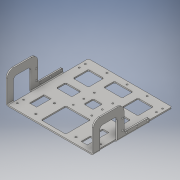
# Autodesk Inventor part: BadanAtasRevisi
Saved by Autodesk Inventor 2016 (Build 200138000, 138)
## iProperties
Created: 2017-04-23
Part Number: BadanAtasRevisi
Material: Generic
Document SubType Name: Modeling
Designer: Ghana
Density: 1 g/cm^3
Appearance: Default
Author: Ghana
Autodesk Inventor part; units mm, degrees
note: some values were not read from the file. Chosen so that the rebuilt part matches the saved one: bend side of "Bend Part6".
ref_plane "YZ Plane" through (0, 0, 0) normal (1, 0, 0) x (0, 1, 0)
ref_plane "XZ Plane" through (0, 0, 0) normal (0, 1, 0) x (-1, 0, 0)
ref_plane "XY Plane" through (0, 0, 0) normal (0, 0, 1) x (1, 0, 0)
sketch "Sketch1" plane through (0, 0, 0) normal (0, 1, 0) x (-1, 0, 0)
  circle A0 centre (82.5, -70) radius 1.3
  circle A1 centre (82.5, -53) radius 1.3
  circle A2 centre (82.5, -87) radius 1.3
  circle A3 centre (100, -125.0019) radius 1.3
  circle A4 centre (35, -125.0019) radius 1.3
  circle A5 centre (52.5, -70) radius 1.3
  circle A6 centre (52.5, -53) radius 1.3
  circle A7 centre (52.5, -87) radius 1.3
  line L0 (85.5, -45.7826) -> (49.5, -45.7826)
  line L1 (47.5, -43.7826) -> (47.5, -7.7826)
  line L2 (49.5, -5.7826) -> (85.5, -5.7826)
  line L3 (87.5, -7.7826) -> (87.5, -43.7826)
  arc A8 (85.5, -45.7826) -> (87.5, -43.7826) centre (85.5, -43.7826) ccw
  arc A9 (47.5, -43.7826) -> (49.5, -45.7826) centre (49.5, -43.7826) ccw
  arc A10 (49.5, -5.7826) -> (47.5, -7.7826) centre (49.5, -7.7826) ccw
  arc A11 (87.5, -7.7826) -> (85.5, -5.7826) centre (85.5, -7.7826) ccw
  line L4 (118, -115) -> (97, -115)
  line L5 (95, -113) -> (95, -92)
  line L6 (97, -90) -> (118, -90)
  line L7 (120, -92) -> (120, -113)
  arc A12 (118, -115) -> (120, -113) centre (118, -113) ccw
  arc A13 (95, -113) -> (97, -115) centre (97, -113) ccw
  arc A14 (97, -90) -> (95, -92) centre (97, -92) ccw
  arc A15 (120, -92) -> (118, -90) centre (118, -92) ccw
  line L8 (17, -115) -> (38, -115)
  line L9 (40, -113) -> (40, -92)
  line L10 (38, -90) -> (17, -90)
  line L11 (15, -92) -> (15, -113)
  arc A16 (15, -113) -> (17, -115) centre (17, -113) ccw
  arc A17 (38, -115) -> (40, -113) centre (38, -113) ccw
  arc A18 (40, -92) -> (38, -90) centre (38, -92) ccw
  arc A19 (17, -90) -> (15, -92) centre (17, -92) ccw
  line L12 (118, -78) -> (97, -78)
  line L13 (95, -76) -> (95, -65)
  line L14 (97, -63) -> (118, -63)
  line L15 (120, -65) -> (120, -76)
  arc A20 (118, -78) -> (120, -76) centre (118, -76) ccw
  arc A21 (95, -76) -> (97, -78) centre (97, -76) ccw
  arc A22 (97, -63) -> (95, -65) centre (97, -65) ccw
  arc A23 (120, -65) -> (118, -63) centre (118, -65) ccw
  line L16 (17, -78) -> (38, -78)
  line L17 (40, -76) -> (40, -65)
  line L18 (38, -63) -> (17, -63)
  line L19 (15, -65) -> (15, -76)
  arc A24 (15, -76) -> (17, -78) centre (17, -76) ccw
  arc A25 (38, -78) -> (40, -76) centre (38, -76) ccw
  arc A26 (40, -65) -> (38, -63) centre (38, -65) ccw
  arc A27 (17, -63) -> (15, -65) centre (17, -65) ccw
  circle A28 centre (100, -40) radius 1.55
  circle A29 centre (100, -10) radius 1.55
  circle A30 centre (35, -40) radius 1.55
  circle A31 centre (35, -10) radius 1.55
  line L20 (120.5, -43.5) -> (109, -43.5)
  line L21 (109, -43.5) -> (109, -20)
  line L22 (109, -20) -> (120.5, -20)
  line L23 (120.5, -20) -> (120.5, -43.5)
  line L24 (15, -43) -> (25, -43)
  line L25 (25, -43) -> (25, -28)
  line L26 (25, -28) -> (15, -28)
  line L27 (15, -28) -> (15, -43)
  line L28 (25, -23) -> (15, -23)
  line L29 (15, -23) -> (15, -8)
  line L30 (15, -8) -> (25, -8)
  line L31 (25, -8) -> (25, -23)
  line L32 (0, 0) -> (135, 0)
  line L33 (135, 0) -> (135, -128)
  line L34 (133, -130) -> (2, -130)
  line L35 (0, -128) -> (0, 0)
  line L36 (62, -62.5) -> (73, -62.5)
  line L37 (75, -64.5) -> (75, -75.5)
  line L38 (73, -77.5) -> (62, -77.5)
  line L39 (60, -75.5) -> (60, -64.5)
  arc A32 (73, -77.5) -> (75, -75.5) centre (73, -75.5) ccw
  arc A33 (60, -75.5) -> (62, -77.5) centre (62, -75.5) ccw
  arc A34 (62, -62.5) -> (60, -64.5) centre (62, -64.5) ccw
  arc A35 (75, -64.5) -> (73, -62.5) centre (73, -64.5) ccw
  circle A36 centre (130, -10) radius 1.3
  circle A37 centre (130, -20) radius 1.3
  circle A38 centre (130, -120) radius 1.3
  circle A39 centre (130, -110) radius 1.3
  line L40 (135, 0) -> (137, 0)
  line L41 (137, 0) -> (137, -10)
  line L42 (137, -90) -> (135, -90)
  line L43 (135, -90) -> (135, 0)
  circle A40 centre (67.5, -125.0019) radius 1.3
  circle A41 centre (139.8, -87) radius 1.3
  circle A42 centre (139.8, -70) radius 1.3
  circle A43 centre (139.8, -53) radius 1.3
  circle A44 centre (146.3, -46.7) radius 1.3
  circle A45 centre (163.3, -46.7) radius 1.3
  line L44 (137, -90) -> (140.4, -90)
  line L45 (142.4, -50.3) -> (142.4, -88)
  line L46 (143.4, -49.3) -> (172.4, -49.3)
  line L47 (182.4, -39.3) -> (182.4, -10)
  line L48 (172.4, 0) -> (137, 0)
  arc A46 (172.4, -49.3) -> (182.4, -39.3) centre (172.4, -39.3) ccw
  arc A47 (182.4, -10) -> (172.4, 0) centre (172.4, -10) ccw
  arc A48 (143.4, -49.3) -> (142.4, -50.3) centre (143.4, -50.3) ccw
  arc A49 (140.4, -90) -> (142.4, -88) centre (140.4, -88) ccw
  arc A50 (133, -130) -> (135, -128) centre (133, -128) ccw
  arc A51 (0, -128) -> (2, -130) centre (2, -128) ccw
  circle A52 centre (5, -10) radius 1.3
  circle A53 centre (5, -20) radius 1.3
  circle A54 centre (5, -120) radius 1.3
  circle A55 centre (5, -110) radius 1.3
  line L49 (0, 0) -> (-2, 0)
  line L50 (-2, 0) -> (-2, -10)
  line L51 (-2, -90) -> (0, -90)
  line L52 (0, -90) -> (0, 0)
  circle A56 centre (-4.8, -87) radius 1.3
  circle A57 centre (-4.8, -70) radius 1.3
  circle A58 centre (-4.8, -53) radius 1.3
  circle A59 centre (-11.3, -46.7) radius 1.3
  circle A60 centre (-28.3, -46.7) radius 1.3
  line L53 (-2, -90) -> (-5.4, -90)
  line L54 (-7.4, -50.3) -> (-7.4, -88)
  line L55 (-8.4, -49.3) -> (-37.4, -49.3)
  line L56 (-47.4, -39.3) -> (-47.4, -10)
  line L57 (-37.4, 0) -> (-2, 0)
  arc A61 (-47.4, -39.3) -> (-37.4, -49.3) centre (-37.4, -39.3) ccw
  arc A62 (-37.4, 0) -> (-47.4, -10) centre (-37.4, -10) ccw
  arc A63 (-7.4, -50.3) -> (-8.4, -49.3) centre (-8.4, -50.3) ccw
  arc A64 (-7.4, -88) -> (-5.4, -90) centre (-5.4, -88) ccw
  line L58 (54.5, -102) -> (80.5, -102)
  line L59 (82.5, -104) -> (82.5, -117.5)
  line L60 (80.5, -119.5) -> (54.5, -119.5)
  line L61 (52.5, -117.5) -> (52.5, -104)
  arc A65 (80.5, -119.5) -> (82.5, -117.5) centre (80.5, -117.5) ccw
  arc A66 (52.5, -117.5) -> (54.5, -119.5) centre (54.5, -117.5) ccw
  arc A67 (54.5, -102) -> (52.5, -104) centre (54.5, -104) ccw
  arc A68 (82.5, -104) -> (80.5, -102) centre (80.5, -104) ccw
  line L62 (67.5, 0) -> (67.5, -34.0355)
  line L63 (135, -10) -> (165, -10)
  line L64 (170, -15) -> (170, -33)
  line L65 (165, -38) -> (135, -38)
  line L66 (135, -38) -> (135, -10)
  arc A69 (165, -38) -> (170, -33) centre (165, -33) ccw
  arc A70 (170, -15) -> (165, -10) centre (165, -15) ccw
  line L67 (137, -38) -> (137, -90)
  line L68 (0, -10) -> (-30, -10)
  line L69 (-35, -15) -> (-35, -33)
  line L70 (-30, -38) -> (0, -38)
  line L71 (0, -38) -> (0, -10)
  arc A71 (-35, -33) -> (-30, -38) centre (-30, -33) ccw
  arc A72 (-30, -10) -> (-35, -15) centre (-30, -15) ccw
  line L72 (-2, -38) -> (-2, -90)
  point P0 (47.5, -5.7826)
  point P1 (47.5, -45.7826)
  point P2 (87.5, -5.7826)
  point P3 (95, -90)
  point P4 (95, -115)
  point P5 (120, -90)
  point P6 (40, -90)
  point P7 (40, -115)
  point P8 (15, -90)
  point P9 (95, -63)
  point P10 (95, -78)
  point P11 (120, -63)
  point P12 (40, -63)
  point P13 (40, -78)
  point P14 (15, -63)
  point P15 (135, -130)
  point P16 (0, -130)
  point P17 (75, -77.5)
  point P18 (75, -62.5)
  point P19 (60, -77.5)
  point P20 (142.4, -49.3)
  point P21 (182.4, -49.3)
  point P22 (-7.4, -49.3)
  point P23 (-47.4, -49.3)
  point P24 (52.5, -102)
  point P25 (82.5, -119.5)
  point P26 (82.5, -102)
  point P27 (170, -38)
  point P28 (170, -10)
  dimension "d28" = 40
  dimension "d29" = 40
  dimension "d30" = 2
  dimension "d33" = 25
  dimension "d34" = 25
  dimension "d52" = 25
  dimension "d53" = 15
  dimension "d61" = 3.1
  dimension "d65" = 11.5
  dimension "d66" = 23.5
  dimension "d70" = 15
  dimension "d71" = 5
  dimension "d72" = 15
  dimension "d115" = 135
  dimension "d116" = 130
  dimension "d117" = 15
  dimension "d118" = 15
  dimension "d119" = 2
  dimension "d122" = 2.6
  dimension "d128" = 2
  dimension "d129" = 10
  dimension "d130" = 2.6
  dimension "d131" = 32.5
  dimension "d132" = 32.5
  dimension "d133" = 65
  dimension "d134" = 30
  dimension "d136" = 2.6
  dimension "d141" = 6.5
  dimension "d143" = 17
  dimension "d144" = 6.3
  dimension "d145" = 17
  dimension "d146" = 17
  dimension "d149" = 40
  dimension "d153" = 10
  dimension "d155" = 1
  dimension "d156" = 2
  dimension "d157" = 2
  dimension "d159" = 15
  dimension "d160" = 17.5
  dimension "d161" = 2
  dimension "d175" = 35
  dimension "d176" = 28
  dimension "d177" = 5
  constraints: 146 end point, 84 point on circle, 73 centre point, 63 point on line, 56 tangent, 32 equal radius, 23 parallel, 14 perpendicular, 13 horizontal, 8 symmetric about line, 5 vertical alignment, 1 horizontal alignment, 1 midpoint, 1 vertical, 2 other
  measures "d28" distance of point (47.5, -5.783) point (87.5, -5.783)
  measures "d29" distance of point (47.5, -45.783) point (47.5, -5.783)
  measures "d30" radius of A8
  measures "d33" distance of point (95, -90) point (120, -90)
  measures "d34" distance of point (95, -115) point (95, -90)
  measures "d52" distance of point (95, -63) point (120, -63)
  measures "d53" distance of point (95, -78) point (95, -63)
  measures "d61" diameter of A28
  measures "d65" distance of L21.end L22.end
  measures "d66" distance of L20.end L21.end
  measures "d70" distance of L25.end L24.end
  measures "d71" distance of L25.end L28.start
  measures "d72" distance of L28.end L29.end
  measures "d115" distance of point (135, -130) point (0, -130)
  measures "d116" distance of L32.end point (135, -130)
  measures "d117" distance of point (75, -77.5) point (60, -77.5)
  measures "d118" distance of point (75, -62.5) point (75, -77.5)
  measures "d119" radius of A32
  measures "d122" diameter of A36
  measures "d128" distance of L42.start L42.end
  measures "d129" distance of L24.start L24.end
  measures "d130" diameter of A3
  measures "d131" distance of A3.centre A40.centre
  measures "d132" distance of A4.centre A40.centre
  measures "d133" distance of A30.centre A28.centre
  measures "d134" distance of A29.centre A28.centre
  measures "d136" diameter of A41
  measures "d141" horizontal distance of A43.centre A44.centre
  measures "d143" distance of A44.centre A45.centre
  measures "d144" vertical distance of A43.centre A44.centre
  measures "d145" distance of A42.centre A41.centre
  measures "d146" distance of A43.centre A42.centre
  measures "d149" distance of point (142.4, -49.3) point (182.4, -49.3)
  measures "d153" radius of A46
  measures "d155" radius of A48
  measures "d156" radius of A49
  measures "d157" radius of A50
  measures "d159" distance of A7.centre point (52.5, -102)
  measures "d160" distance of point (82.5, -102) point (82.5, -119.5)
  measures "d161" radius of A65
  measures "d175" distance of point (170, -38) L65.end
  measures "d176" distance of point (170, -10) point (170, -38)
  measures "d177" radius of A69
extrude "Extrusion5" add sketch "Sketch1" along normal blind 2 contours L32 L33 A50 L34 A51 L35 | L35 L68 L50 L49 | L50 L68 A72 L69 A71 L70 L72 L53 A64 L54 A63 L55 A61 L56 A62 L57 | L40 L41 L63 L33 | L35 L51 L72 L70 | L48 A47 L47 A46 L46 A48 L45 A49 L44 L67 L65 A69 L64 A70 L63 L41 | L65 L67 L42 L33
sketch "Sketch7" plane through (0, 2, 0) normal (0, 1, 0) x (1, 0, 0)
  arc A0 (-47.5, 43.7826) -> (-49.5, 45.7826) centre (-49.5, 43.7826) ccw projected
  line L0 (-47.5, 43.7826) -> (-47.5, 7.7826) projected
  arc A1 (-49.5, 5.7826) -> (-47.5, 7.7826) centre (-49.5, 7.7826) ccw projected
  line L1 (-49.5, 5.7826) -> (-85.5, 5.7826) projected
  arc A2 (-87.5, 7.7826) -> (-85.5, 5.7826) centre (-85.5, 7.7826) ccw projected
  line L2 (-87.5, 7.7826) -> (-87.5, 43.7826) projected
  arc A3 (-85.5, 45.7826) -> (-87.5, 43.7826) centre (-85.5, 43.7826) ccw projected
  line L3 (-85.5, 45.7826) -> (-49.5, 45.7826) projected
  arc A4 (-15, 113) -> (-17, 115) centre (-17, 113) ccw projected
  line L4 (-15, 113) -> (-15, 92) projected
  arc A5 (-17, 90) -> (-15, 92) centre (-17, 92) ccw projected
  line L5 (-17, 90) -> (-38, 90) projected
  arc A6 (-40, 92) -> (-38, 90) centre (-38, 92) ccw projected
  line L6 (-40, 92) -> (-40, 113) projected
  arc A7 (-38, 115) -> (-40, 113) centre (-38, 113) ccw projected
  line L7 (-38, 115) -> (-17, 115) projected
  arc A8 (-95, 113) -> (-97, 115) centre (-97, 113) ccw projected
  line L8 (-95, 113) -> (-95, 92) projected
  arc A9 (-97, 90) -> (-95, 92) centre (-97, 92) ccw projected
  line L9 (-97, 90) -> (-118, 90) projected
  arc A10 (-120, 92) -> (-118, 90) centre (-118, 92) ccw projected
  line L10 (-120, 92) -> (-120, 113) projected
  arc A11 (-118, 115) -> (-120, 113) centre (-118, 113) ccw projected
  line L11 (-118, 115) -> (-97, 115) projected
  arc A12 (-52.5, 117.5) -> (-54.5, 119.5) centre (-54.5, 117.5) ccw projected
  line L12 (-52.5, 117.5) -> (-52.5, 104) projected
  arc A13 (-54.5, 102) -> (-52.5, 104) centre (-54.5, 104) ccw projected
  line L13 (-54.5, 102) -> (-80.5, 102) projected
  arc A14 (-82.5, 104) -> (-80.5, 102) centre (-80.5, 104) ccw projected
  line L14 (-82.5, 104) -> (-82.5, 117.5) projected
  arc A15 (-80.5, 119.5) -> (-82.5, 117.5) centre (-80.5, 117.5) ccw projected
  line L15 (-80.5, 119.5) -> (-54.5, 119.5) projected
  arc A16 (-38, 78) -> (-40, 76) centre (-38, 76) ccw projected
  line L16 (-38, 78) -> (-17, 78) projected
  arc A17 (-15, 76) -> (-17, 78) centre (-17, 76) ccw projected
  line L17 (-15, 76) -> (-15, 65) projected
  arc A18 (-17, 63) -> (-15, 65) centre (-17, 65) ccw projected
  line L18 (-17, 63) -> (-38, 63) projected
  arc A19 (-40, 65) -> (-38, 63) centre (-38, 65) ccw projected
  line L19 (-40, 65) -> (-40, 76) projected
  arc A20 (-95, 76) -> (-97, 78) centre (-97, 76) ccw projected
  line L20 (-95, 76) -> (-95, 65) projected
  arc A21 (-97, 63) -> (-95, 65) centre (-97, 65) ccw projected
  line L21 (-97, 63) -> (-118, 63) projected
  arc A22 (-120, 65) -> (-118, 63) centre (-118, 65) ccw projected
  line L22 (-120, 65) -> (-120, 76) projected
  arc A23 (-118, 78) -> (-120, 76) centre (-118, 76) ccw projected
  line L23 (-118, 78) -> (-97, 78) projected
  line L24 (-109, 43.5) -> (-109, 20) projected
  line L25 (-109, 20) -> (-120.5, 20) projected
  line L26 (-120.5, 20) -> (-120.5, 43.5) projected
  line L27 (-120.5, 43.5) -> (-109, 43.5) projected
  arc A24 (-60, 75.5) -> (-62, 77.5) centre (-62, 75.5) ccw projected
  line L28 (-60, 75.5) -> (-60, 64.5) projected
  arc A25 (-62, 62.5) -> (-60, 64.5) centre (-62, 64.5) ccw projected
  line L29 (-62, 62.5) -> (-73, 62.5) projected
  arc A26 (-75, 64.5) -> (-73, 62.5) centre (-73, 64.5) ccw projected
  line L30 (-75, 64.5) -> (-75, 75.5) projected
  arc A27 (-73, 77.5) -> (-75, 75.5) centre (-73, 75.5) ccw projected
  line L31 (-73, 77.5) -> (-62, 77.5) projected
  line L32 (-15, 23) -> (-15, 8) projected
  line L33 (-15, 8) -> (-25, 8) projected
  line L34 (-25, 8) -> (-25, 23) projected
  line L35 (-25, 23) -> (-15, 23) projected
  line L36 (-15, 43) -> (-15, 28) projected
  line L37 (-15, 28) -> (-25, 28) projected
  line L38 (-25, 28) -> (-25, 43) projected
  line L39 (-25, 43) -> (-15, 43) projected
  circle A28 centre (-35, 10) radius 1.55 projected
  circle A29 centre (-35, 40) radius 1.55 projected
  circle A30 centre (-100, 10) radius 1.55 projected
  circle A31 centre (-100, 40) radius 1.55 projected
  circle A32 centre (-5, 110) radius 1.3 projected
  circle A33 centre (-5, 120) radius 1.3 projected
  circle A34 centre (-5, 10) radius 1.3 projected
  circle A35 centre (-5, 20) radius 1.3 projected
  circle A36 centre (-67.5, 125.0019) radius 1.3 projected
  circle A37 centre (-130, 110) radius 1.3 projected
  circle A38 centre (-130, 120) radius 1.3 projected
  circle A39 centre (-130, 20) radius 1.3 projected
  circle A40 centre (-130, 10) radius 1.3 projected
  circle A41 centre (-52.5, 70) radius 1.3 projected
  circle A42 centre (-52.5, 53) radius 1.3 projected
  circle A43 centre (-52.5, 87) radius 1.3 projected
  circle A44 centre (-35, 125.0019) radius 1.3 projected
  circle A45 centre (-100, 125.0019) radius 1.3 projected
  circle A46 centre (-82.5, 87) radius 1.3 projected
  circle A47 centre (-82.5, 53) radius 1.3 projected
  circle A48 centre (-82.5, 70) radius 1.3 projected
  circle A49 centre (-163.3, 46.7) radius 1.3 projected
  circle A50 centre (-146.3, 46.7) radius 1.3 projected
  circle A51 centre (-139.8, 53) radius 1.3 projected
  circle A52 centre (-139.8, 70) radius 1.3 projected
  circle A53 centre (-139.8, 87) radius 1.3 projected
  circle A54 centre (28.3, 46.7) radius 1.3 projected
  circle A55 centre (11.3, 46.7) radius 1.3 projected
  circle A56 centre (4.8, 53) radius 1.3 projected
  circle A57 centre (4.8, 70) radius 1.3 projected
  circle A58 centre (4.8, 87) radius 1.3 projected
  line L40 (0, 10) -> (0, 38) projected
  line L41 (0, 38) -> (30, 38) projected
  arc A59 (35, 33) -> (30, 38) centre (30, 33) ccw projected
  line L42 (35, 33) -> (35, 15) projected
  arc A60 (30, 10) -> (35, 15) centre (30, 15) ccw projected
  line L43 (30, 10) -> (0, 10) projected
  line L44 (-135, 10) -> (-165, 10) projected
  arc A61 (-170, 15) -> (-165, 10) centre (-165, 15) ccw projected
  line L45 (-170, 15) -> (-170, 33) projected
  arc A62 (-165, 38) -> (-170, 33) centre (-165, 33) ccw projected
  line L46 (-165, 38) -> (-135, 38) projected
  line L47 (-135, 38) -> (-135, 10) projected
  line L48 (-172.4, 0) -> (37.4, 0) projected
  arc A63 (37.4, 0) -> (47.4, 10) centre (37.4, 10) ccw projected
  line L49 (47.4, 10) -> (47.4, 39.3) projected
  arc A64 (47.4, 39.3) -> (37.4, 49.3) centre (37.4, 39.3) ccw projected
  line L50 (37.4, 49.3) -> (8.4, 49.3) projected
  arc A65 (7.4, 50.3) -> (8.4, 49.3) centre (8.4, 50.3) ccw projected
  line L51 (7.4, 50.3) -> (7.4, 88) projected
  arc A66 (7.4, 88) -> (5.4, 90) centre (5.4, 88) ccw projected
  line L52 (5.4, 90) -> (0, 90) projected
  line L53 (0, 90) -> (0, 128) projected
  arc A67 (0, 128) -> (-2, 130) centre (-2, 128) ccw projected
  line L54 (-2, 130) -> (-133, 130) projected
  arc A68 (-133, 130) -> (-135, 128) centre (-133, 128) ccw projected
  line L55 (-135, 128) -> (-135, 90) projected
  line L56 (-135, 90) -> (-140.4, 90) projected
  arc A69 (-140.4, 90) -> (-142.4, 88) centre (-140.4, 88) ccw projected
  line L57 (-142.4, 88) -> (-142.4, 50.3) projected
  arc A70 (-143.4, 49.3) -> (-142.4, 50.3) centre (-143.4, 50.3) ccw projected
  line L58 (-143.4, 49.3) -> (-172.4, 49.3) projected
  arc A71 (-172.4, 49.3) -> (-182.4, 39.3) centre (-172.4, 39.3) ccw projected
  line L59 (-182.4, 39.3) -> (-182.4, 10) projected
  arc A72 (-182.4, 10) -> (-172.4, 0) centre (-172.4, 10) ccw projected
  line L60 (-135, 90) -> (-135, 0)
  point P0 (0, 0)
  constraints: 2 end point, 1 perpendicular, 1 point on line
bend part "Bend Part5" radius 1.2732 angle 90 line through (-135, 2, -90) along (0, 0, 1) centre toward (0, 1, 0) moving side (-1, 0, 0) both sides no
sketch "Sketch8" plane through (0, 2, 0) normal (0, 1, 0) x (1, 0, 0)
  line L0 (-135, 0) -> (-135, 10) projected
  line L1 (-135, 0) -> (37.4, 0) projected
  arc A0 (37.4, 0) -> (47.4, 10) centre (37.4, 10) ccw projected
  line L2 (47.4, 10) -> (47.4, 39.3) projected
  arc A1 (47.4, 39.3) -> (37.4, 49.3) centre (37.4, 39.3) ccw projected
  line L3 (37.4, 49.3) -> (8.4, 49.3) projected
  arc A2 (7.4, 50.3) -> (8.4, 49.3) centre (8.4, 50.3) ccw projected
  line L4 (7.4, 50.3) -> (7.4, 88) projected
  arc A3 (7.4, 88) -> (5.4, 90) centre (5.4, 88) ccw projected
  line L5 (5.4, 90) -> (0, 90) projected
  line L6 (0, 90) -> (0, 128) projected
  arc A4 (0, 128) -> (-2, 130) centre (-2, 128) ccw projected
  line L7 (-2, 130) -> (-133, 130) projected
  arc A5 (-133, 130) -> (-135, 128) centre (-133, 128) ccw projected
  line L8 (-135, 128) -> (-135, 90) projected
  line L9 (-135, 38) -> (-135, 90) projected
  line L10 (-135, 38) -> (-135, 10) projected
  line L11 (0, 10) -> (0, 38) projected
  line L12 (0, 38) -> (30, 38) projected
  arc A6 (35, 33) -> (30, 38) centre (30, 33) ccw projected
  line L13 (35, 33) -> (35, 15) projected
  arc A7 (30, 10) -> (35, 15) centre (30, 15) ccw projected
  line L14 (30, 10) -> (0, 10) projected
  circle A8 centre (4.8, 87) radius 1.3 projected
  circle A9 centre (4.8, 70) radius 1.3 projected
  circle A10 centre (4.8, 53) radius 1.3 projected
  circle A11 centre (11.3, 46.7) radius 1.3 projected
  circle A12 centre (28.3, 46.7) radius 1.3 projected
  circle A13 centre (-82.5, 70) radius 1.3 projected
  circle A14 centre (-82.5, 53) radius 1.3 projected
  circle A15 centre (-82.5, 87) radius 1.3 projected
  circle A16 centre (-100, 125.0019) radius 1.3 projected
  circle A17 centre (-35, 125.0019) radius 1.3 projected
  circle A18 centre (-52.5, 87) radius 1.3 projected
  circle A19 centre (-52.5, 53) radius 1.3 projected
  circle A20 centre (-52.5, 70) radius 1.3 projected
  circle A21 centre (-130, 10) radius 1.3 projected
  circle A22 centre (-130, 20) radius 1.3 projected
  circle A23 centre (-130, 120) radius 1.3 projected
  circle A24 centre (-130, 110) radius 1.3 projected
  circle A25 centre (-67.5, 125.0019) radius 1.3 projected
  circle A26 centre (-5, 20) radius 1.3 projected
  circle A27 centre (-5, 10) radius 1.3 projected
  circle A28 centre (-5, 120) radius 1.3 projected
  circle A29 centre (-5, 110) radius 1.3 projected
  circle A30 centre (-100, 40) radius 1.55 projected
  circle A31 centre (-100, 10) radius 1.55 projected
  circle A32 centre (-35, 40) radius 1.55 projected
  circle A33 centre (-35, 10) radius 1.55 projected
  line L15 (-15, 43) -> (-15, 28) projected
  line L16 (-15, 28) -> (-25, 28) projected
  line L17 (-25, 28) -> (-25, 43) projected
  line L18 (-25, 43) -> (-15, 43) projected
  line L19 (-15, 23) -> (-15, 8) projected
  line L20 (-15, 8) -> (-25, 8) projected
  line L21 (-25, 8) -> (-25, 23) projected
  line L22 (-25, 23) -> (-15, 23) projected
  arc A34 (-60, 75.5) -> (-62, 77.5) centre (-62, 75.5) ccw projected
  line L23 (-60, 75.5) -> (-60, 64.5) projected
  arc A35 (-62, 62.5) -> (-60, 64.5) centre (-62, 64.5) ccw projected
  line L24 (-62, 62.5) -> (-73, 62.5) projected
  arc A36 (-75, 64.5) -> (-73, 62.5) centre (-73, 64.5) ccw projected
  line L25 (-75, 64.5) -> (-75, 75.5) projected
  arc A37 (-73, 77.5) -> (-75, 75.5) centre (-73, 75.5) ccw projected
  line L26 (-73, 77.5) -> (-62, 77.5) projected
  line L27 (-109, 43.5) -> (-109, 20) projected
  line L28 (-109, 20) -> (-120.5, 20) projected
  line L29 (-120.5, 20) -> (-120.5, 43.5) projected
  line L30 (-120.5, 43.5) -> (-109, 43.5) projected
  arc A38 (-95, 76) -> (-97, 78) centre (-97, 76) ccw projected
  line L31 (-95, 76) -> (-95, 65) projected
  arc A39 (-97, 63) -> (-95, 65) centre (-97, 65) ccw projected
  line L32 (-97, 63) -> (-118, 63) projected
  arc A40 (-120, 65) -> (-118, 63) centre (-118, 65) ccw projected
  line L33 (-120, 65) -> (-120, 76) projected
  arc A41 (-118, 78) -> (-120, 76) centre (-118, 76) ccw projected
  line L34 (-118, 78) -> (-97, 78) projected
  arc A42 (-38, 78) -> (-40, 76) centre (-38, 76) ccw projected
  line L35 (-38, 78) -> (-17, 78) projected
  arc A43 (-15, 76) -> (-17, 78) centre (-17, 76) ccw projected
  line L36 (-15, 76) -> (-15, 65) projected
  arc A44 (-17, 63) -> (-15, 65) centre (-17, 65) ccw projected
  line L37 (-17, 63) -> (-38, 63) projected
  arc A45 (-40, 65) -> (-38, 63) centre (-38, 65) ccw projected
  line L38 (-40, 65) -> (-40, 76) projected
  arc A46 (-52.5, 117.5) -> (-54.5, 119.5) centre (-54.5, 117.5) ccw projected
  line L39 (-52.5, 117.5) -> (-52.5, 104) projected
  arc A47 (-54.5, 102) -> (-52.5, 104) centre (-54.5, 104) ccw projected
  line L40 (-54.5, 102) -> (-80.5, 102) projected
  arc A48 (-82.5, 104) -> (-80.5, 102) centre (-80.5, 104) ccw projected
  line L41 (-82.5, 104) -> (-82.5, 117.5) projected
  arc A49 (-80.5, 119.5) -> (-82.5, 117.5) centre (-80.5, 117.5) ccw projected
  line L42 (-80.5, 119.5) -> (-54.5, 119.5) projected
  arc A50 (-95, 113) -> (-97, 115) centre (-97, 113) ccw projected
  line L43 (-95, 113) -> (-95, 92) projected
  arc A51 (-97, 90) -> (-95, 92) centre (-97, 92) ccw projected
  line L44 (-97, 90) -> (-118, 90) projected
  arc A52 (-120, 92) -> (-118, 90) centre (-118, 92) ccw projected
  line L45 (-120, 92) -> (-120, 113) projected
  arc A53 (-118, 115) -> (-120, 113) centre (-118, 113) ccw projected
  line L46 (-118, 115) -> (-97, 115) projected
  arc A54 (-15, 113) -> (-17, 115) centre (-17, 113) ccw projected
  line L47 (-15, 113) -> (-15, 92) projected
  arc A55 (-17, 90) -> (-15, 92) centre (-17, 92) ccw projected
  line L48 (-17, 90) -> (-38, 90) projected
  arc A56 (-40, 92) -> (-38, 90) centre (-38, 92) ccw projected
  line L49 (-40, 92) -> (-40, 113) projected
  arc A57 (-38, 115) -> (-40, 113) centre (-38, 113) ccw projected
  line L50 (-38, 115) -> (-17, 115) projected
  arc A58 (-47.5, 43.7826) -> (-49.5, 45.7826) centre (-49.5, 43.7826) ccw projected
  line L51 (-47.5, 43.7826) -> (-47.5, 7.7826) projected
  arc A59 (-49.5, 5.7826) -> (-47.5, 7.7826) centre (-49.5, 7.7826) ccw projected
  line L52 (-49.5, 5.7826) -> (-85.5, 5.7826) projected
  arc A60 (-87.5, 7.7826) -> (-85.5, 5.7826) centre (-85.5, 7.7826) ccw projected
  line L53 (-87.5, 7.7826) -> (-87.5, 43.7826) projected
  arc A61 (-85.5, 45.7826) -> (-87.5, 43.7826) centre (-85.5, 43.7826) ccw projected
  line L54 (-85.5, 45.7826) -> (-49.5, 45.7826) projected
  line L55 (0, 90) -> (0, 0)
  constraints: 2 end point, 1 vertical
bend part "Bend Part6" radius 1.2732 angle 90 line through (0, 2, -90) along (0, 0, 1) centre toward (0, 1, 0) moving side (1, 0, 0) both sides no
body "Solid4"
